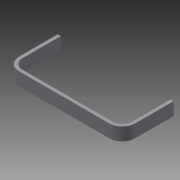
# Autodesk Inventor part: Generic brace
Saved by Autodesk Inventor 2013 (Build 170138000, 138)
## iProperties
Created: 2013-01-20
Part Number: Generic brace
Material: Generic
Document SubType Name: Sheet Metal
Designer: Arpan
Density: 1 g/cm^3
Sheet Metal Rule: Default
Author: Arpan
Autodesk Inventor part; units mm, degrees
ref_plane "YZ Plane" through (0, 0, 0) normal (1, 0, 0) x (0, 1, 0)
ref_plane "XZ Plane" through (0, 0, 0) normal (0, 1, 0) x (-1, 0, 0)
ref_plane "XY Plane" through (0, 0, 0) normal (0, 0, 1) x (1, 0, 0)
sketch "Sketch1" plane through (0, 0, 0) normal (0, 0, 1) x (1, 0, 0)
  line L0 (0, 0) -> (-114.3, 0)
  line L1 (-114.3, 0) -> (-114.3, 12.7)
  line L2 (-114.3, 12.7) -> (0, 12.7)
  line L3 (0, 12.7) -> (0, 0)
  dimension "d0" = 114.3
  dimension "d1" = 12.7
  measures "d0" distance of L0.start L0.end
  measures "d1" distance of L0.end L1.end
extrude "Plate1" add sketch "Sketch1" along normal blind 3.048
sketch "Sketch2" plane through (-3.048, 0, 3.048) normal (1, 0, 0) x (0, 1, 0)
  line L0 (12.7, 0) -> (0, 0)
  line L1 (0, 0) -> (0, -50.673)
  line L2 (0, -50.673) -> (12.7, -50.673)
  line L3 (12.7, -50.673) -> (12.7, 0)
  constraints: 6 end point, 1 horizontal, 1 perpendicular, 1 vertical
edge flange "Flange1" height 47.625 angle 90 thickness 3.048 bend radius 9.525 thickness toward (1, 0, 0) relief straight relief width 3.048 relief depth 1.524 edges at (0, 6.35, 0) wall of the first edge with corners at (-3.048, 12.7, 3.048) (-3.048, 0, 3.048) (-3.048, 0, -47.625) (-3.048, 12.7, -47.625)
bend "Bend1"
corner "Corner1"
sketch "Sketch3" plane through (-111.252, 12.7, 3.048) normal (-1, 0, 0) x (0, -1, 0)
  line L0 (12.7, 0) -> (0, 0)
  line L1 (0, 0) -> (0, -50.673)
  line L2 (0, -50.673) -> (12.7, -50.673)
  line L3 (12.7, -50.673) -> (12.7, 0)
  constraints: 6 end point, 1 horizontal, 1 perpendicular, 1 vertical
edge flange "Flange2" height 47.625 angle 90 thickness 3.048 bend radius 9.525 thickness toward (-1, 0, 0) relief straight relief width 3.048 relief depth 1.524 edges at (-114.3, 6.35, 0) wall of the first edge with corners at (-111.252, 0, 3.048) (-111.252, 12.7, 3.048) (-111.252, 12.7, -47.625) (-111.252, 0, -47.625)
bend "Bend2"
corner "Corner2"
equation "\"d3\" = BendReliefWidth"
equation "\"d4\" = BendReliefDepth"
equation "\"d5\" = MinimumRemnant"
equation "\"d6\" = BendRadius"
equation "\"d10\" = CornerReliefSize"
equation "\"d11\" = GapSize"
equation "\"d12\" = JacobiRadiusSize"
equation "\"d13\" = BendReliefWidth"
equation "\"d14\" = BendReliefDepth"
equation "\"d15\" = MinimumRemnant"
equation "\"d16\" = BendRadius"
equation "\"d20\" = CornerReliefSize"
equation "\"d21\" = GapSize"
equation "\"d22\" = JacobiRadiusSize"
equation "\"BendRadius\" = Thickness"
equation "\"BendReliefWidth\" = Thickness"
equation "\"BendReliefDepth\" = 0.5 * Thickness"
equation "\"CornerReliefSize\" = 4 * Thickness"
equation "\"MinimumRemnant\" = 2 * Thickness"
equation "\"TransitionRadius\" = BendRadius"
equation "\"JacobiRadiusSize\" = BendRadius"
equation "\"GapSize\" = Thickness"
equation "\"d2\" = BendRadius"
equation "\"Thickness\" = 3.048"
body "Solid1"
